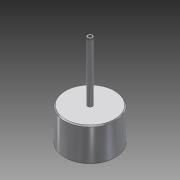
# Autodesk Inventor part: Fixture_Weight
Saved by Autodesk Inventor 2015 (Build 190159000, 159)
## iProperties
Created: 2014-12-16
Part Number: Fixture_Weight
Material: Generic
Document SubType Name: Modeling
Designer: amarschn
Density: 1 g/cm^3
Appearance: Aluminum - Dark
Author: amarschn
Autodesk Inventor part; units mm, degrees
ref_plane "YZ Plane" through (0, 0, 0) normal (1, 0, 0) x (0, 1, 0)
ref_plane "XZ Plane" through (0, 0, 0) normal (0, 1, 0) x (-1, 0, 0)
ref_plane "XY Plane" through (0, 0, 0) normal (0, 0, 1) x (1, 0, 0)
sketch "Sketch2" plane through (0, 0, 0) normal (1, 0, 0) x (0, 1, 0)
  line L0 (0, 0) -> (0, -31.496)
  line L1 (0, -31.496) -> (41.275, -31.496)
  line L2 (41.275, -31.496) -> (41.275, -3.175)
  line L3 (114.554, -3.175) -> (114.554, 0)
  line L4 (114.554, 0) -> (0, 0)
  line L5 (113.284, -3.175) -> (113.284, -2.921)
  line L6 (113.284, -2.921) -> (112.649, -2.921)
  line L7 (112.649, -2.921) -> (112.649, -3.175)
  line L8 (41.275, -3.175) -> (112.649, -3.175)
  line L9 (113.284, -3.175) -> (114.554, -3.175)
  dimension "d0" = 41.275
  dimension "d1" = 73.279
  dimension "d2" = 31.496
  dimension "d18" = 1.27
  dimension "d19" = 0.635
  dimension "d20" = 0.254
  dimension "d21" = 3.175
  constraints: 20 end point, 10 perpendicular, 2 point on line, 2 vertical, 1 collinear
  measures "d0" distance between parallel lines of L2 L0
  measures "d1" distance of L2.end L3.start
  measures "d2" distance of L4.end L0.end
  measures "d18" distance between parallel lines of L3 L5
  measures "d19" distance between parallel lines of L7 L5
  measures "d20" distance between parallel lines of L6 L9
  measures "d21" distance between parallel lines of L4 L9
revolve "Revolution1" add sketch "Sketch2" angle 360 about axis through (0, 114.554, 0) along (0, -1, 0)
chamfer "Chamfer1" distance 1.27 angle 45 2 edges at (0, 41.275, 31.496) (0, 0, 31.496)
sketch "Sketch3" plane through (0, 114.554, 0) normal (0, 1, 0) x (1, 0, 0)
  point P0 (0, 0)
  point P1 (0, 0)
  constraints: 1 coincident
hole "Hole1" at (0, 114.554, 0) direction (0, -1, 0) diameter 3.9624 depth 25.4 tip angle 118 thread size "10-32 UNF" class "2B" standard "ANSI Unified Screw Threads"
sketch "Sketch4" plane through (0, 0, 0) normal (0, -1, 0) x (1, 0, 0)
  circle A0 centre (0, 0) radius 3.175 projected
  constraints: 1 coincident
hole "Hole2" at (0, 0, 0) direction (0, 1, 0) diameter 3.302 depth 10.922 tip angle 118 thread size "8-32 UNC" class "2B" standard "ANSI Unified Screw Threads"
body "Solid1"
